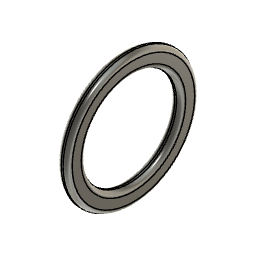
Valve outlet spacer (Autodesk Fusion 360 design; units mm, degrees)
Autodesk Fusion 360 part; units mm, degrees
sketch "Sketch1" plane through (0, 0, 0) normal (1, 0, 0) x (0, 1, 0)
  circle A0 centre (0, 0) radius 10.5
  circle A1 centre (0, 0) radius 14.5
  dimension "d1" = 21
  dimension "d2" = 29
  constraint coincident A0.centre A1.centre
  constraint concentric A0 A1
  measures "d1" diameter of A0
  measures "d2" diameter of A1
extrude "Extrude1" add sketch "Sketch1" along normal blind 2.4
fillet "Fillet1" radius 1 2 faces at (2.4, 13.0736, -1.242) (0, 13.0736, -1.242)
